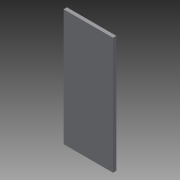
# Autodesk Inventor part: docisk do mostka
Saved by Autodesk Inventor 2015 (Build 190159000, 159)
## iProperties
Created: 2015-05-04
Part Number: docisk do mostka
Material: Ogólny
Document SubType Name: Modeling
Designer: Kuba
Density: 1 g/cm^3
Appearance: Domyślna
Author: Kuba
Autodesk Inventor part; units mm, degrees
ref_plane "YZ Plane" through (0, 0, 0) normal (1, 0, 0) x (0, 1, 0)
ref_plane "XZ Plane" through (0, 0, 0) normal (0, 1, 0) x (-1, 0, 0)
ref_plane "XY Plane" through (0, 0, 0) normal (0, 0, 1) x (1, 0, 0)
sketch "Szkic1" plane through (0, 0, 0) normal (0, 1, 0) x (-1, 0, 0)
  line L0 (-15, -35.5) -> (15, -35.5)
  line L1 (15, -35.5) -> (15, 35.5)
  line L2 (15, 35.5) -> (-15, 35.5)
  line L3 (-15, 35.5) -> (-15, -35.5)
  line L4 (-15, -35.5) -> (15, 35.5) construction
  line L5 (15, -35.5) -> (-15, 35.5) construction
  point P0 (0, 0)
  dimension "d0" = 30
  dimension "d1" = 71
  constraints: 12 end point, 2 midpoint, 2 parallel, 1 horizontal, 1 perpendicular
  measures "d0" distance of L2.end L1.end
  measures "d1" distance of L1.end L0.end
extrude "Wyciągnięcie proste1" add sketch "Szkic1" along normal blind 2
sketch "Szkic2" plane through (0, 0, 0) normal (0, -1, 0) x (1, 0, 0)
  circle A0 centre (11, 0) radius 1.5 projected
  circle A1 centre (19, -31.5) radius 1.5 projected
  circle A2 centre (-11, 31.5) radius 1.5 projected
  circle A3 centre (-11, -31.5) radius 1.5 projected
  circle A4 centre (19, 31.5) radius 1.5 projected
  circle A5 centre (-11, 0) radius 1.5 projected
  line L0 (23.5, -35.5) -> (-15.5, -35.5) projected
  line L1 (23.5, 35.5) -> (23.5, -35.5) projected
  line L2 (-15.5, 35.5) -> (23.5, 35.5) projected
  line L3 (-15.5, -35.5) -> (-15.5, 35.5) projected
  point P0 (0, 0)
hole "Otwór1" at (11, 0, 0) at (-11, 0, 0) at (-11, 0, 31.5) at (-11, 0, -31.5) direction (0, 1, 0) diameter 3.5 end through all
